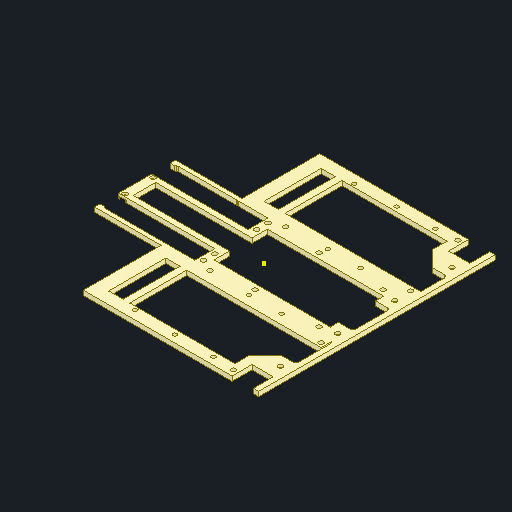
# Autodesk Inventor part: base
Saved by Autodesk Inventor 2023 (Build 270158000, 158)
## iProperties
Created: 2024-04-29
Part Number: base
Material: Nylon 6/6
Document SubType Name: Modeling
Designer: szymo
Density: 1.13 g/cm^3
Appearance: Nylon 6
Mass: 38.5341 g
Surface Area: 286.672 cm^2
Volume: 34.1009 cm^3
Author: szymo
Autodesk Inventor part; units mm, degrees
ref_plane "YZ Plane" through (0, 0, 0) normal (1, 0, 0) x (0, 1, 0)
ref_plane "XZ Plane" through (0, 0, 0) normal (0, 1, 0) x (-1, 0, 0)
ref_plane "XY Plane" through (0, 0, 0) normal (0, 0, 1) x (1, 0, 0)
sketch "Sketch1" plane through (0, 0, 0) normal (0, 1, 0) x (-1, 0, 0)
  line L0 (99, 89) -> (-99, 89)
  line L1 (-99, 89) -> (-99, -89)
  line L2 (-99, -89) -> (99, -89)
  line L3 (99, -89) -> (99, 89)
  line L4 (99, 89) -> (-99, -89) construction
  line L5 (-99, 89) -> (99, -89) construction
  line L6 (-99, 89) -> (-85, 89)
  line L7 (-85, 89) -> (-85, -89)
  line L8 (-85, -89) -> (-99, -89)
  line L9 (-99, -89) -> (-99, 89)
  line L10 (99, 89) -> (97, 89)
  line L11 (97, 89) -> (97, -89)
  line L12 (97, -89) -> (99, -89)
  line L13 (99, -89) -> (99, 89)
  line L14 (97, 33) -> (97, 35)
  line L15 (97, -33) -> (97, -35)
  line L16 (97, 32.8) -> (97, 35)
  line L17 (97, -32.8) -> (97, -35)
  line L18 (97, 89) -> (47, 89)
  line L19 (47, 89) -> (47, 30.5)
  line L20 (47, 30.5) -> (97, 30.5)
  line L21 (97, 30.5) -> (97, 89)
  line L22 (97, -89) -> (47, -89)
  line L23 (47, -89) -> (47, -30.5)
  line L24 (47, -30.5) -> (97, -30.5)
  line L25 (97, -30.5) -> (97, -89)
  line L26 (-81, 74) -> (-81, 89) projected
  line L27 (-81, 31) -> (-81, 55) projected
  line L28 (-81, -12) -> (-81, 12) projected
  line L29 (-81, -55) -> (-81, -31) projected
  line L30 (-81, -89) -> (-81, -74) projected
  arc A0 (-81, 74) -> (-79, 72) centre (-79, 74) ccw projected
  line L31 (-70, 72) -> (-79, 72) projected
  line L32 (-70, 57) -> (-70, 72) projected
  line L33 (-79, 57) -> (-70, 57) projected
  arc A1 (-79, 57) -> (-81, 55) centre (-79, 55) ccw projected
  arc A2 (-81, 31) -> (-79, 29) centre (-79, 31) ccw projected
  line L34 (-70, 29) -> (-79, 29) projected
  line L35 (-70, 14) -> (-70, 29) projected
  line L36 (-79, 14) -> (-70, 14) projected
  arc A3 (-79, 14) -> (-81, 12) centre (-79, 12) ccw projected
  arc A4 (-81, -12) -> (-79, -14) centre (-79, -12) ccw projected
  line L37 (-70, -14) -> (-79, -14) projected
  line L38 (-70, -29) -> (-70, -14) projected
  line L39 (-79, -29) -> (-70, -29) projected
  arc A5 (-79, -29) -> (-81, -31) centre (-79, -31) ccw projected
  arc A6 (-81, -55) -> (-79, -57) centre (-79, -55) ccw projected
  line L40 (-70, -57) -> (-79, -57) projected
  line L41 (-70, -72) -> (-70, -57) projected
  line L42 (-79, -72) -> (-70, -72) projected
  arc A7 (-79, -72) -> (-81, -74) centre (-79, -74) ccw projected
  circle A8 centre (-77, -64.5) radius 1.2295 projected
  circle A9 centre (-77, -21.5) radius 1.2295 projected
  circle A10 centre (-77, 21.5) radius 1.2295 projected
  circle A11 centre (-77, 64.5) radius 1.2295 projected
  line L43 (-65, 89) -> (-79, 89)
  line L44 (-79, 89) -> (-79, 75)
  line L45 (-79, 75) -> (-65, 75)
  line L46 (-65, 75) -> (-65, 89)
  line L47 (-65, 89) -> (-81, 89)
  line L48 (-81, 89) -> (-81, 74)
  line L49 (-81, 74) -> (-65, 74)
  line L50 (-65, 74) -> (-65, 89)
  line L51 (-99, 0) -> (97, 0)
  line L52 (0, 0) -> (-99, 0) construction
  line L53 (-65, -89) -> (-79, -89)
  line L54 (-79, -89) -> (-79, -75)
  line L55 (-79, -75) -> (-65, -75)
  line L56 (-65, -75) -> (-65, -89)
  line L57 (-65, -89) -> (-81, -89)
  line L58 (-81, -89) -> (-81, -74)
  line L59 (-81, -74) -> (-65, -74)
  line L60 (-65, -74) -> (-65, -89)
  line L61 (77.5, 29.5) -> (66.5, 29.5) projected
  line L62 (66.5, -29.5) -> (77.5, -29.5) projected
  point P0 (47, 89)
  point P1 (47, -89)
  point P2 (97, -30.5)
  point P3 (97, 30.5)
  point P4 (-81, -89)
  point P5 (-79, -74)
  dimension "d0" = 198
  dimension "d1" = 178
  dimension "d2" = 14
  dimension "d3" = 2
  dimension "d16" = 50
  dimension "d17" = 58.5
  dimension "d18" = 50
  dimension "d19" = 58.5
  dimension "d22" = 14
  dimension "d23" = 14
  dimension "d24" = 2
  dimension "d25" = 1
  dimension "d26" = 2
  dimension "d87" = 1
  dimension "d88" = 1
  constraints: 88 end point, 14 parallel, 10 symmetric about line, 8 perpendicular, 8 point on line, 7 horizontal, 4 midpoint, 2 collinear
  measures "d0" distance of L2.end L1.end
  measures "d1" distance of L1.end L0.end
  measures "d2" distance of L7.end L8.end
  measures "d3" distance of L12.end L11.end
  measures "d16" distance of L20.end L19.end
  measures "d17" distance of L19.end L18.end
  measures "d18" distance of L23.end L24.end
  measures "d19" distance of L22.end L23.end
  measures "d22" distance of L45.end L44.end
  measures "d23" distance of L44.end L43.end
  measures "d24" distance between parallel lines of L26 L44
  measures "d25" distance between parallel lines of L45 L49
  measures "d26" distance between parallel lines of L31 L49
  measures "d87" distance between parallel lines of L20 L61
  measures "d88" distance between parallel lines of L24 L62
extrude "Extrusion1" add sketch "Sketch1" along normal blind 3.5 contours L19 L20 L11 L51 L28 A3 L36 L35 L34 A2 L27 A1 L33 L32 L31 A0 L49 L50 L46 L0 | L2 L56 L60 L59 A7 L42 L41 L40 A6 L29 A5 L39 L38 L37 A4 L28 L51 L11 L24 L23 | L26 A0 L31 L32 L33 A1 L27 A2 L34 L35 L36 A3 L28 L51 L7 L0 | L28 A4 L37 L38 L39 A5 L29 A6 L40 L41 L42 A7 L30 L2 L7 L51 | A8 | A9 | A10 | A11
sketch "Sketch9" plane through (0, 0, 0) normal (0, -1, 0) x (1, 0, 0)
  circle A0 centre (-94, -10.5) radius 1.4 projected
  circle A1 centre (-94, 10.5) radius 1.4 projected
  circle A2 centre (-21.25, -24.25) radius 1.8 projected
  circle A3 centre (-21.25, -15.75) radius 1.8 projected
  circle A4 centre (-21.25, 15.75) radius 1.8 projected
  circle A5 centre (-21.25, 24.25) radius 1.8 projected
  circle A6 centre (-12.1414, 28.5) radius 1.8 projected
  circle A7 centre (-12.1414, -28.5) radius 1.8 projected
  circle A8 centre (17.4, -24.1) radius 1.6 projected
  circle A9 centre (17.4, 24.1) radius 1.6 projected
  circle A10 centre (65.6, 24.1) radius 1.6 projected
  circle A11 centre (65.6, -24.1) radius 1.6 projected
  circle A12 centre (76.75, -33.75) radius 1.8 projected
  circle A13 centre (76.75, 33.75) radius 1.8 projected
  circle A14 centre (61.5, 84.5) radius 1.8 projected
  circle A15 centre (61.5, -84.5) radius 1.8 projected
  point P0 (0, 0)
  constraints: 16 coincident
hole "m3" at (-94, 0, -10.5) at (-94, 0, 10.5) at (61.5, 0, -84.5) at (61.5, 0, 84.5) at (76.75, 0, 33.75) at (65.6, 0, 24.1) at (65.6, 0, -24.1) at (76.75, 0, -33.75) at (17.4, 0, 24.1) at (17.4, 0, -24.1) at (-12.1414, 0, -28.5) at (-21.25, 0, -24.25) at (-21.25, 0, -15.75) at (-21.25, 0, 15.75) at (-21.25, 0, 24.25) at (-12.1414, 0, 28.5) direction (0, 1, 0) diameter 3.6 end through all counterbore diameter 11 counterbore depth 0 clearance for "Hex Head Cap Screw ISO 24014 (Spotface)" size "M3" standard "ISO"
sketch "Sketch10" plane through (0, 0, 0) normal (0, -1, 0) x (1, 0, 0)
  circle A0 centre (61.5, -84.5) radius 1.8 projected
  circle A1 centre (76.75, -33.75) radius 1.8 projected
  circle A2 centre (65.6, -24.1) radius 1.8 projected
  circle A3 centre (65.6, 24.1) radius 1.8 projected
  circle A4 centre (76.75, 33.75) radius 1.8 projected
  circle A5 centre (61.5, 84.5) radius 1.8 projected
  circle A6 centre (17.4, 24.1) radius 1.8 projected
  circle A7 centre (17.4, -24.1) radius 1.8 projected
  circle A8 centre (-12.1414, -28.5) radius 1.8 projected
  circle A9 centre (-21.25, -24.25) radius 1.8 projected
  circle A10 centre (-21.25, -15.75) radius 1.8 projected
  circle A11 centre (-21.25, 15.75) radius 1.8 projected
  circle A12 centre (-21.25, 24.25) radius 1.8 projected
  circle A13 centre (-12.1414, 28.5) radius 1.8 projected
  circle A14 centre (-94, 10.5) radius 1.8 projected
  circle A15 centre (-94, -10.5) radius 1.8 projected
  line L0 (-94, -7.2668) -> (-91.2, -8.8834)
  line L1 (-91.2, -8.8834) -> (-91.2, -12.1166)
  line L2 (-91.2, -12.1166) -> (-94, -13.7332)
  line L3 (-94, -13.7332) -> (-96.8, -12.1166)
  line L4 (-96.8, -12.1166) -> (-96.8, -8.8834)
  line L5 (-96.8, -8.8834) -> (-94, -7.2668)
  line L6 (-94, 13.7332) -> (-91.2, 12.1166)
  line L7 (-91.2, 12.1166) -> (-91.2, 8.8834)
  line L8 (-91.2, 8.8834) -> (-94, 7.2668)
  line L9 (-94, 7.2668) -> (-96.8, 8.8834)
  line L10 (-96.8, 8.8834) -> (-96.8, 12.1166)
  line L11 (-96.8, 12.1166) -> (-94, 13.7332)
  point P0 (0, 0)
  dimension "d96" = 5.6
  dimension "d98" = 5.6
  constraints: 24 end point, 2 coincident, 26 other
  measures "d96" distance between parallel lines of L4 L1
  measures "d98" distance between parallel lines of L7 L10
extrude "m3_nut" cut sketch "Sketch10" against normal blind 1.6 contours L0 L1 L2 L3 L4 L5 | L6 L7 L8 L9 L10 L11
sketch "Sketch11" plane through (0, 0, 0) normal (0, -1, 0) x (1, 0, 0)
  circle A0 centre (-14.5, -82.4087) radius 1.15 projected
  circle A1 centre (16.5, -83.5) radius 1.15 projected
  circle A2 centre (45.4385, -83.5) radius 1.15 projected
  circle A3 centre (45.4385, 83.5) radius 1.15 projected
  circle A4 centre (16.5, 83.5) radius 1.15 projected
  circle A5 centre (-14.5, 82.4087) radius 1.15 projected
  circle A6 centre (18.4119, 29.75) radius 1.55 projected
  circle A7 centre (43.009, 29.75) radius 1.55 projected
  circle A8 centre (43.009, -29.75) radius 1.55 projected
  circle A9 centre (18.4119, -29.75) radius 1.55 projected
  point P0 (0, 0)
  constraints: 10 coincident
hole "m2.5" at (-14.5, 0, -82.4087) at (-14.5, 0, 82.4087) at (16.5, 0, 83.5) at (45.4385, 0, 83.5) at (43.009, 0, 29.75) at (18.4119, 0, 29.75) at (18.4119, 0, -29.75) at (43.009, 0, -29.75) at (45.4385, 0, -83.5) at (16.5, 0, -83.5) direction (0, 1, 0) diameter 3.1 end through all clearance for "Countersunk Flat Head Screw ISO 2009/7046" size "M2.5" standard "ISO"
sketch "m2.5_nut" plane through (0, 0, 0) normal (0, -1, 0) x (1, 0, 0)
  circle A0 centre (-14.5, -82.4087) radius 1.55 projected
  circle A1 centre (16.5, -83.5) radius 1.55 projected
  circle A2 centre (45.4385, -83.5) radius 1.55 projected
  circle A3 centre (45.4385, 83.5) radius 1.55 projected
  circle A4 centre (16.5, 83.5) radius 1.55 projected
  circle A5 centre (-14.5, 82.4087) radius 1.55 projected
  circle A6 centre (18.4119, -29.75) radius 1.55 projected
  circle A7 centre (43.009, -29.75) radius 1.55 projected
  circle A8 centre (43.009, 29.75) radius 1.55 projected
  circle A9 centre (18.4119, 29.75) radius 1.55 projected
  point P0 (0, 0)
sketch "Sketch13" plane through (0, 0, 0) normal (0, -1, 0) x (1, 0, 0)
  circle A0 centre (77, 21.5) radius 1.2295 projected
  circle A1 centre (77, -64.5) radius 1.2295 projected
  circle A2 centre (77, -21.5) radius 1.2295 projected
  circle A3 centre (77, 64.5) radius 1.2295 projected
  line L0 (79, -72) -> (70, -72) projected
  line L1 (70, -72) -> (70, -57) projected
  line L2 (70, -57) -> (79, -57) projected
  arc A4 (79, -57) -> (81, -55) centre (79, -55) ccw projected
  line L3 (81, -55) -> (81, -31) projected
  arc A5 (81, -31) -> (79, -29) centre (79, -31) ccw projected
  line L4 (79, -29) -> (70, -29) projected
  line L5 (70, -29) -> (70, -14) projected
  line L6 (70, -14) -> (79, -14) projected
  arc A6 (79, -14) -> (81, -12) centre (79, -12) ccw projected
  line L7 (81, -12) -> (81, 12) projected
  arc A7 (81, 12) -> (79, 14) centre (79, 12) ccw projected
  line L8 (79, 14) -> (70, 14) projected
  line L9 (70, 14) -> (70, 29) projected
  line L10 (70, 29) -> (79, 29) projected
  arc A8 (79, 29) -> (81, 31) centre (79, 31) ccw projected
  line L11 (81, 31) -> (81, 55) projected
  arc A9 (81, 55) -> (79, 57) centre (79, 55) ccw projected
  line L12 (79, 57) -> (70, 57) projected
  line L13 (70, 57) -> (70, 72) projected
  line L14 (70, 72) -> (79, 72) projected
  arc A10 (79, 72) -> (81, 74) centre (79, 74) ccw projected
  line L15 (81, 74) -> (81, 89) projected
  line L16 (85, 89) -> (81, 89) projected
  line L17 (85, -89) -> (85, 89) projected
  line L18 (85, -89) -> (81, -89) projected
  line L19 (81, -89) -> (81, -74) projected
  arc A11 (81, -74) -> (79, -72) centre (79, -74) ccw projected
  point P0 (0, 0)
  constraints: 4 coincident
hole "Hole6" at (77, 0, -64.5) at (77, 0, -21.5) at (77, 0, 21.5) at (77, 0, 64.5) direction (0, 1, 0) diameter 3.6 end through all countersink diameter 7 countersink angle 90
sketch "Sketch14" plane through (0, 3.5, 0) normal (0, -1, 0) x (1, 0, 0)
  circle A0 centre (70, -83) radius 1.75
  line L0 (14.0482, -86) -> (-12.0482, -86)
  arc A1 (-12.0482, -86) -> (-12, -85.6932) centre (-13, -85.6932) ccw
  line L1 (-12, -85.6932) -> (-12, -80.9087)
  arc A2 (-12, -80.9087) -> (-13, -79.9087) centre (-13, -80.9087) ccw
  line L2 (-13, -79.9087) -> (-16, -79.9087)
  arc A3 (-16, -79.9087) -> (-17, -80.9087) centre (-16, -80.9087) ccw
  line L3 (-17, -80.9087) -> (-17, -86)
  line L4 (-17, -86) -> (-21.8397, -86)
  arc A4 (-22.8397, -85) -> (-21.8397, -86) centre (-21.8397, -85) ccw
  line L5 (-22.8397, -85) -> (-22.8397, -81.6)
  line L6 (-22.8397, -81.6) -> (-31.5, -81.6)
  line L7 (-31.5, -81.6) -> (-40.1603, -81.6)
  line L8 (-40.1603, -85) -> (-40.1603, -81.6)
  arc A5 (-41.1603, -86) -> (-40.1603, -85) centre (-41.1603, -85) ccw
  line L9 (-41.1603, -86) -> (-47, -86)
  line L10 (-47, -89) -> (-47, -86)
  line L11 (-47, -89) -> (80, -89)
  line L12 (80, -89) -> (80, -88)
  line L13 (80, -88) -> (78.75, -88)
  arc A6 (74.5, -83.75) -> (78.75, -88) centre (78.75, -83.75) ccw
  line L14 (74.5, -83.75) -> (74.5, -80.25)
  arc A7 (74.5, -80.25) -> (70.25, -76) centre (70.25, -80.25) ccw
  line L15 (70.25, -76) -> (68.2269, -76)
  line L16 (68.2269, -76) -> (68.2269, -75.875)
  arc A8 (65, -71.75) -> (68.2269, -75.875) centre (69.25, -71.75) ccw
  line L17 (65, -71.75) -> (65, -69)
  line L18 (65, -69) -> (58, -69)
  line L19 (58, -69) -> (58, -74)
  line L20 (58, -74) -> (58, -86)
  line L21 (58, -86) -> (47.8903, -86)
  arc A9 (47.8903, -86) -> (47.9385, -85.6932) centre (46.9385, -85.6932) ccw
  line L22 (47.9385, -85.6932) -> (47.9385, -82)
  arc A10 (47.9385, -82) -> (46.9385, -81) centre (46.9385, -82) ccw
  line L23 (46.9385, -81) -> (43.9385, -81)
  arc A11 (43.9385, -81) -> (42.9385, -82) centre (43.9385, -82) ccw
  line L24 (42.9385, -82) -> (42.9385, -85.6932)
  arc A12 (42.9385, -85.6932) -> (42.9867, -86) centre (43.9385, -85.6932) ccw
  line L25 (42.9867, -86) -> (18.9518, -86)
  arc A13 (18.9518, -86) -> (19, -85.6932) centre (18, -85.6932) ccw
  line L26 (19, -85.6932) -> (19, -82)
  arc A14 (19, -82) -> (18, -81) centre (18, -82) ccw
  line L27 (18, -81) -> (15, -81)
  arc A15 (15, -81) -> (14, -82) centre (15, -82) ccw
  line L28 (14, -82) -> (14, -85.6932)
  arc A16 (14, -85.6932) -> (14.0482, -86) centre (15, -85.6932) ccw
  circle A17 centre (16.5, -83.5) radius 1.15
  circle A18 centre (-14.5, -82.4087) radius 1.15
  circle A19 centre (45.4385, -83.5) radius 1.15
  circle A20 centre (61.5, -84.5) radius 1.8
  circle A21 centre (18.4119, -29.75) radius 1.55
  circle A22 centre (43.009, -29.75) radius 1.55
  circle A23 centre (17.4, -24.1) radius 1.6
  circle A24 centre (65.6, -24.1) radius 1.6
  circle A25 centre (-12.1414, -28.5) radius 1.8
  circle A26 centre (76.75, -33.75) radius 1.8
  arc A27 (69.6, -27.9275) -> (73.5136, -30.785) centre (72.6, -27.9275) ccw
  line L29 (69.6, -27.9275) -> (69.6, -20.1)
  line L30 (69.6, -20.1) -> (61.6, -20.1)
  line L31 (61.6, -20.1) -> (61.6, -27)
  arc A28 (56.6, -32) -> (61.6, -27) centre (56.6, -27) ccw
  line L32 (56.6, -32) -> (53.1217, -32)
  arc A29 (47.3676, -27.7) -> (53.1217, -32) centre (53.1217, -26) ccw
  line L33 (47.3676, -27.7) -> (38.6504, -27.7)
  arc A30 (32.8963, -32) -> (38.6504, -27.7) centre (32.8963, -26) ccw
  line L34 (32.8963, -32) -> (28.5247, -32)
  arc A31 (22.7705, -27.7) -> (28.5247, -32) centre (28.5247, -26) ccw
  line L35 (22.7705, -27.7) -> (22.7705, -20.1)
  line L36 (22.7705, -20.1) -> (14.0533, -20.1)
  line L37 (14.0533, -20.1) -> (14.0533, -27.7)
  arc A32 (8.2992, -32) -> (14.0533, -27.7) centre (8.2992, -26) ccw
  line L38 (8.2992, -32) -> (-0.7828, -32)
  arc A33 (-7.7828, -25) -> (-0.7828, -32) centre (-0.7828, -25) ccw
  line L39 (-7.7828, -25) -> (-16.5, -25)
  line L40 (-16.5, -28) -> (-16.5, -25)
  arc A34 (-20.5, -32) -> (-16.5, -28) centre (-20.5, -28) ccw
  line L41 (-20.5, -32) -> (-47, -32)
  line L42 (-47, -37) -> (-47, -32)
  line L43 (-47, -37) -> (52.4519, -37)
  line L44 (52.4519, -36) -> (52.4519, -37)
  line L45 (52.4519, -37) -> (80, -37)
  line L46 (80, -37) -> (80, -30.5)
  line L47 (80, -30.5) -> (75.3408, -30.5)
  arc A35 (75.3408, -30.5) -> (73.5136, -30.785) centre (75.3408, -36.5) ccw
  circle A36 centre (18.4119, 29.75) radius 1.55
  circle A37 centre (43.009, 29.75) radius 1.55
  circle A38 centre (17.4, 24.1) radius 1.6
  circle A39 centre (65.6, 24.1) radius 1.6
  circle A40 centre (-12.1414, 28.5) radius 1.8
  circle A41 centre (76.75, 33.75) radius 1.8
  arc A42 (73.5136, 30.785) -> (69.6, 27.9275) centre (72.6, 27.9275) ccw
  arc A43 (73.5136, 30.785) -> (75.3408, 30.5) centre (75.3408, 36.5) ccw
  line L48 (80, 30.5) -> (75.3408, 30.5)
  line L49 (80, 37) -> (80, 30.5)
  line L50 (52.4519, 37) -> (80, 37)
  line L51 (52.4519, 36) -> (52.4519, 37)
  line L52 (-47, 37) -> (52.4519, 37)
  line L53 (-47, 37) -> (-47, 32)
  line L54 (-20.5, 32) -> (-47, 32)
  arc A44 (-16.5, 28) -> (-20.5, 32) centre (-20.5, 28) ccw
  line L55 (-16.5, 28) -> (-16.5, 25)
  line L56 (-7.7828, 25) -> (-16.5, 25)
  arc A45 (-0.7828, 32) -> (-7.7828, 25) centre (-0.7828, 25) ccw
  line L57 (8.2992, 32) -> (-0.7828, 32)
  arc A46 (14.0533, 27.7) -> (8.2992, 32) centre (8.2992, 26) ccw
  line L58 (14.0533, 20.1) -> (14.0533, 27.7)
  line L59 (22.7705, 20.1) -> (14.0533, 20.1)
  line L60 (22.7705, 27.7) -> (22.7705, 20.1)
  arc A47 (28.5247, 32) -> (22.7705, 27.7) centre (28.5247, 26) ccw
  line L61 (32.8963, 32) -> (28.5247, 32)
  arc A48 (38.6504, 27.7) -> (32.8963, 32) centre (32.8963, 26) ccw
  line L62 (47.3676, 27.7) -> (38.6504, 27.7)
  arc A49 (53.1217, 32) -> (47.3676, 27.7) centre (53.1217, 26) ccw
  line L63 (56.6, 32) -> (53.1217, 32)
  arc A50 (61.6, 27) -> (56.6, 32) centre (56.6, 27) ccw
  line L64 (61.6, 20.1) -> (61.6, 27)
  line L65 (69.6, 20.1) -> (61.6, 20.1)
  line L66 (69.6, 27.9275) -> (69.6, 20.1)
  line L67 (14.0482, 86) -> (-12.0482, 86)
  arc A51 (14.0482, 86) -> (14, 85.6932) centre (15, 85.6932) ccw
  line L68 (14, 82) -> (14, 85.6932)
  arc A52 (14, 82) -> (15, 81) centre (15, 82) ccw
  line L69 (18, 81) -> (15, 81)
  arc A53 (18, 81) -> (19, 82) centre (18, 82) ccw
  line L70 (19, 85.6932) -> (19, 82)
  arc A54 (19, 85.6932) -> (18.9518, 86) centre (18, 85.6932) ccw
  line L71 (42.9867, 86) -> (18.9518, 86)
  arc A55 (42.9867, 86) -> (42.9385, 85.6932) centre (43.9385, 85.6932) ccw
  line L72 (42.9385, 82) -> (42.9385, 85.6932)
  arc A56 (42.9385, 82) -> (43.9385, 81) centre (43.9385, 82) ccw
  line L73 (46.9385, 81) -> (43.9385, 81)
  arc A57 (46.9385, 81) -> (47.9385, 82) centre (46.9385, 82) ccw
  line L74 (47.9385, 85.6932) -> (47.9385, 82)
  arc A58 (47.9385, 85.6932) -> (47.8903, 86) centre (46.9385, 85.6932) ccw
  line L75 (58, 86) -> (47.8903, 86)
  line L76 (58, 74) -> (58, 86)
  line L77 (58, 69) -> (58, 74)
  line L78 (65, 69) -> (58, 69)
  line L79 (65, 71.75) -> (65, 69)
  arc A59 (68.2269, 75.875) -> (65, 71.75) centre (69.25, 71.75) ccw
  line L80 (68.2269, 76) -> (68.2269, 75.875)
  line L81 (70.25, 76) -> (68.2269, 76)
  arc A60 (70.25, 76) -> (74.5, 80.25) centre (70.25, 80.25) ccw
  line L82 (74.5, 83.75) -> (74.5, 80.25)
  arc A61 (78.75, 88) -> (74.5, 83.75) centre (78.75, 83.75) ccw
  line L83 (80, 88) -> (78.75, 88)
  line L84 (80, 89) -> (80, 88)
  line L85 (-47, 89) -> (80, 89)
  line L86 (-47, 89) -> (-47, 86)
  line L87 (-41.1603, 86) -> (-47, 86)
  arc A62 (-40.1603, 85) -> (-41.1603, 86) centre (-41.1603, 85) ccw
  line L88 (-40.1603, 85) -> (-40.1603, 81.6)
  line L89 (-31.5, 81.6) -> (-40.1603, 81.6)
  line L90 (-22.8397, 81.6) -> (-31.5, 81.6)
  line L91 (-22.8397, 85) -> (-22.8397, 81.6)
  arc A63 (-21.8397, 86) -> (-22.8397, 85) centre (-21.8397, 85) ccw
  line L92 (-17, 86) -> (-21.8397, 86)
  line L93 (-17, 80.9087) -> (-17, 86)
  arc A64 (-17, 80.9087) -> (-16, 79.9087) centre (-16, 80.9087) ccw
  line L94 (-13, 79.9087) -> (-16, 79.9087)
  arc A65 (-13, 79.9087) -> (-12, 80.9087) centre (-13, 80.9087) ccw
  line L95 (-12, 85.6932) -> (-12, 80.9087)
  arc A66 (-12, 85.6932) -> (-12.0482, 86) centre (-13, 85.6932) ccw
  circle A67 centre (16.5, 83.5) radius 1.15
  circle A68 centre (-14.5, 82.4087) radius 1.15
  circle A69 centre (45.4385, 83.5) radius 1.15
  circle A70 centre (70, 80) radius 1.75
  circle A71 centre (61.5, 84.5) radius 1.8
  line L96 (-24.5, 21) -> (-24.5, 27.5)
  line L97 (-18, 21) -> (-24.5, 21)
  line L98 (-18, 30.5) -> (-18, 21)
  line L99 (-97, 30.5) -> (-18, 30.5)
  line L100 (-97, 30.5) -> (-97, 26.5)
  line L101 (-93.7321, 26.5) -> (-97, 26.5)
  arc A72 (-93.7321, 26.5) -> (-92.866, 27) centre (-93.7321, 27.5) ccw
  arc A73 (-92, 27.5) -> (-92.866, 27) centre (-92, 26.5) ccw
  line L102 (-78.8409, 27.5) -> (-92, 27.5)
  spline S0 degree 3 poles (-75.7417, 26) (-75.7753, 26.0631) (-75.8128, 26.1246) (-76.0566, 26.4695) (-76.3938, 26.7337) (-77.0078, 27.0936) (-77.4015, 27.2556) (-78.0794, 27.4407) (-78.4928, 27.5) (-78.8409, 27.5) knots 0 0 0 0 0.058061 0.058061 0.375369 0.375369 0.690666 0.690666 1 1 1 1
  line L103 (-68.2583, 26) -> (-75.7417, 26)
  spline S1 degree 3 poles (-68.2583, 26) (-68.2382, 26.0379) (-68.2174, 26.0746) (-68.0344, 26.3642) (-67.7636, 26.6069) (-67.1915, 26.9981) (-66.7665, 27.1943) (-66.018, 27.4248) (-65.5523, 27.5) (-65.1591, 27.5) knots 0 0 0 0 0.035027 0.035027 0.30423 0.30423 0.650773 0.650773 1 1 1 1
  line L104 (-47.8217, 27.5) -> (-65.1591, 27.5)
  spline S2 degree 3 poles (-45.6477, 26) (-45.6733, 26.0786) (-45.7018, 26.1547) (-45.8425, 26.4593) (-46.0302, 26.7067) (-46.4247, 27.0666) (-46.7063, 27.2391) (-47.2204, 27.4381) (-47.5457, 27.5) (-47.8217, 27.5) knots 0 0 0 0 0.086487 0.086487 0.378353 0.378353 0.688736 0.688736 1 1 1 1
  line L105 (-38.9709, 26) -> (-45.6477, 26)
  spline S3 degree 3 poles (-38.9709, 26) (-38.9452, 26.0786) (-38.9168, 26.1547) (-38.7761, 26.4593) (-38.5883, 26.7067) (-38.1939, 27.0666) (-37.9122, 27.2391) (-37.3982, 27.4381) (-37.0728, 27.5) (-36.7968, 27.5) knots 0 0 0 0 0.086487 0.086487 0.378353 0.378353 0.688736 0.688736 1 1 1 1
  line L106 (-24.5, 27.5) -> (-36.7968, 27.5)
  circle A74 centre (-21.25, 24.25) radius 1.8
  circle A75 centre (-94, 10.5) radius 1.4
  circle A76 centre (-21.25, 15.75) radius 1.8
  line L107 (-37.4639, 12.5) -> (-24, 12.5)
  spline S4 degree 3 poles (-38.9709, 13) (-38.7801, 12.8633) (-38.5578, 12.7418) (-38.085, 12.5634) (-37.7489, 12.5) (-37.4639, 12.5) knots 0 0 0 0 0.435873 0.435873 1 1 1 1
  line L108 (-38.9709, 13) -> (-41.358, 13)
  spline S5 degree 3 poles (-43.2606, 13) (-43.1675, 13) (-43.0559, 12.9938) (-42.7588, 12.9716) (-42.5141, 12.9484) (-42.1044, 12.9484) (-41.8597, 12.9716) (-41.5626, 12.9938) (-41.4511, 13) (-41.358, 13) knots 0 0 0 0 0.156235 0.156235 0.5 0.5 0.843765 0.843765 1 1 1 1
  line L109 (-43.2606, 13) -> (-45.6477, 13)
  spline S6 degree 3 poles (-45.6477, 13) (-45.8385, 12.8633) (-46.0608, 12.7418) (-46.5335, 12.5634) (-46.8696, 12.5) (-47.1547, 12.5) knots 0 0 0 0 0.435873 0.435873 1 1 1 1
  line L110 (-67.6471, 12.5) -> (-47.1547, 12.5)
  line L111 (-70.9629, 12.5) -> (-67.6471, 12.5)
  line L112 (-72, 12.5) -> (-70.9629, 12.5)
  line L113 (-73.0371, 12.5) -> (-72, 12.5)
  line L114 (-76.3529, 12.5) -> (-73.0371, 12.5)
  line L115 (-97, 12.5) -> (-76.3529, 12.5)
  line L116 (-97, 8.5) -> (-97, 12.5)
  line L117 (-97, 8.5) -> (-17.5, 8.5)
  line L118 (-17.5, 8.5) -> (-17.5, 19)
  line L119 (-24, 19) -> (-17.5, 19)
  line L120 (-24, 12.5) -> (-24, 19)
  circle A77 centre (-94, -10.5) radius 1.4
  circle A78 centre (-21.25, -15.75) radius 1.8
  line L121 (-37.4639, -12.5) -> (-24, -12.5)
  line L122 (-24, -12.5) -> (-24, -19)
  line L123 (-24, -19) -> (-17.5, -19)
  line L124 (-17.5, -8.5) -> (-17.5, -19)
  line L125 (-97, -8.5) -> (-17.5, -8.5)
  line L126 (-97, -8.5) -> (-97, -12.5)
  line L127 (-97, -12.5) -> (-76.3529, -12.5)
  line L128 (-76.3529, -12.5) -> (-73.0371, -12.5)
  line L129 (-73.0371, -12.5) -> (-72, -12.5)
  line L130 (-72, -12.5) -> (-70.9629, -12.5)
  line L131 (-70.9629, -12.5) -> (-67.6471, -12.5)
  line L132 (-67.6471, -12.5) -> (-47.1547, -12.5)
  spline S7 degree 3 poles (-45.6477, -13) (-45.8385, -12.8633) (-46.0608, -12.7418) (-46.5335, -12.5634) (-46.8696, -12.5) (-47.1547, -12.5) knots 0 0 0 0 0.435873 0.435873 1 1 1 1
  line L133 (-43.2606, -13) -> (-45.6477, -13)
  spline S8 degree 3 poles (-43.2606, -13) (-43.1675, -13) (-43.0559, -12.9938) (-42.7588, -12.9716) (-42.5141, -12.9484) (-42.1044, -12.9484) (-41.8597, -12.9716) (-41.5626, -12.9938) (-41.4511, -13) (-41.358, -13) knots 0 0 0 0 0.156235 0.156235 0.5 0.5 0.843765 0.843765 1 1 1 1
  line L134 (-38.9709, -13) -> (-41.358, -13)
  spline S9 degree 3 poles (-38.9709, -13) (-38.7801, -12.8633) (-38.5578, -12.7418) (-38.085, -12.5634) (-37.7489, -12.5) (-37.4639, -12.5) knots 0 0 0 0 0.435873 0.435873 1 1 1 1
  line L135 (-24.5, -21) -> (-24.5, -27.5)
  line L136 (-24.5, -27.5) -> (-36.7968, -27.5)
  spline S10 degree 3 poles (-38.9709, -26) (-38.9452, -26.0786) (-38.9168, -26.1547) (-38.7761, -26.4593) (-38.5883, -26.7067) (-38.1939, -27.0666) (-37.9122, -27.2391) (-37.3982, -27.4381) (-37.0728, -27.5) (-36.7968, -27.5) knots 0 0 0 0 0.086487 0.086487 0.378353 0.378353 0.688736 0.688736 1 1 1 1
  line L137 (-38.9709, -26) -> (-45.6477, -26)
  spline S11 degree 3 poles (-45.6477, -26) (-45.6733, -26.0786) (-45.7018, -26.1547) (-45.8425, -26.4593) (-46.0302, -26.7067) (-46.4247, -27.0666) (-46.7063, -27.2391) (-47.2204, -27.4381) (-47.5457, -27.5) (-47.8217, -27.5) knots 0 0 0 0 0.086487 0.086487 0.378353 0.378353 0.688736 0.688736 1 1 1 1
  line L138 (-47.8217, -27.5) -> (-65.1591, -27.5)
  spline S12 degree 3 poles (-68.2583, -26) (-68.2382, -26.0379) (-68.2174, -26.0746) (-68.0344, -26.3642) (-67.7636, -26.6069) (-67.1915, -26.9981) (-66.7665, -27.1943) (-66.018, -27.4248) (-65.5523, -27.5) (-65.1591, -27.5) knots 0 0 0 0 0.035027 0.035027 0.30423 0.30423 0.650773 0.650773 1 1 1 1
  line L139 (-68.2583, -26) -> (-75.7417, -26)
  spline S13 degree 3 poles (-75.7417, -26) (-75.7753, -26.0631) (-75.8128, -26.1246) (-76.0566, -26.4695) (-76.3938, -26.7337) (-77.0078, -27.0936) (-77.4015, -27.2556) (-78.0794, -27.4407) (-78.4928, -27.5) (-78.8409, -27.5) knots 0 0 0 0 0.058061 0.058061 0.375369 0.375369 0.690666 0.690666 1 1 1 1
  line L140 (-78.8409, -27.5) -> (-92, -27.5)
  arc A79 (-92.866, -27) -> (-92, -27.5) centre (-92, -26.5) ccw
  arc A80 (-92.866, -27) -> (-93.7321, -26.5) centre (-93.7321, -27.5) ccw
  line L141 (-93.7321, -26.5) -> (-97, -26.5)
  line L142 (-97, -30.5) -> (-97, -26.5)
  line L143 (-97, -30.5) -> (-18, -30.5)
  line L144 (-18, -30.5) -> (-18, -21)
  line L145 (-18, -21) -> (-24.5, -21)
  circle A81 centre (-21.25, -24.25) radius 1.8
  line L146 (-22, -8.5) -> (-22, 8.5)
  line L147 (-22, 8.5) -> (-90, 8.5)
  line L148 (-90, 8.5) -> (-90, -8.5)
  line L149 (-90, -8.5) -> (-22, -8.5)
  line L150 (-15.5, -70.1149) -> (50.5, -70.1149)
  line L151 (50.5, -70.1149) -> (50.5, -40.1149)
  line L152 (-15.5, -40.1149) -> (50.5, -40.1149)
  line L153 (-15.5, -70.1149) -> (-15.5, -40.1149)
  line L154 (50.5, 71.1831) -> (-15.5, 71.1831)
  line L155 (-15.5, 71.1831) -> (-15.5, 41.1831)
  line L156 (50.5, 41.1831) -> (-15.5, 41.1831)
  line L157 (50.5, 71.1831) -> (50.5, 41.1831)
  line L158 (-36.8852, -42) -> (-31.5, -42)
  line L159 (-31.5, -42) -> (-26.1148, -42)
  line L160 (-26.1148, -42) -> (-26.1148, -69.7)
  line L161 (-26.1148, -69.7) -> (-36.8852, -69.7)
  line L162 (-36.8852, -69.7) -> (-36.8852, -42)
  line L163 (-26.1148, 42) -> (-31.5, 42)
  line L164 (-31.5, 42) -> (-36.8852, 42)
  line L165 (-36.8852, 42) -> (-36.8852, 69.7)
  line L166 (-36.8852, 69.7) -> (-26.1148, 69.7)
  line L167 (-26.1148, 69.7) -> (-26.1148, 42)
  line L168 (85, -89) -> (99, -89)
  line L169 (99, -89) -> (99, 89)
  line L170 (85, 89) -> (99, 89)
  line L171 (85, -89) -> (85, 89)
  circle A82 centre (77, 21.5) radius 1.2295
  circle A83 centre (77, -64.5) radius 1.2295
  circle A84 centre (77, -21.5) radius 1.2295
  circle A85 centre (77, 64.5) radius 1.2295
  line L172 (70, -72) -> (79, -72)
  arc A86 (81, -74) -> (79, -72) centre (79, -74) ccw
  line L173 (81, -74) -> (81, -89)
  line L174 (81, -89) -> (85, -89)
  line L175 (85, -89) -> (85, 89)
  line L176 (81, 89) -> (85, 89)
  line L177 (81, 89) -> (81, 74)
  arc A87 (79, 72) -> (81, 74) centre (79, 74) ccw
  line L178 (79, 72) -> (70, 72)
  line L179 (70, 57) -> (70, 72)
  line L180 (70, 57) -> (79, 57)
  arc A88 (81, 55) -> (79, 57) centre (79, 55) ccw
  line L181 (81, 55) -> (81, 31)
  arc A89 (79, 29) -> (81, 31) centre (79, 31) ccw
  line L182 (79, 29) -> (70, 29)
  line L183 (70, 14) -> (70, 29)
  line L184 (70, 14) -> (79, 14)
  arc A90 (81, 12) -> (79, 14) centre (79, 12) ccw
  line L185 (81, 12) -> (81, -12)
  arc A91 (79, -14) -> (81, -12) centre (79, -12) ccw
  line L186 (79, -14) -> (70, -14)
  line L187 (70, -29) -> (70, -14)
  line L188 (70, -29) -> (79, -29)
  arc A92 (81, -31) -> (79, -29) centre (79, -31) ccw
  line L189 (81, -31) -> (81, -55)
  arc A93 (79, -57) -> (81, -55) centre (79, -55) ccw
  line L190 (79, -57) -> (70, -57)
  line L191 (70, -72) -> (70, -57)
  line L192 (81, -89) -> (81, -74)
  line L193 (81, -74) -> (65, -74)
  line L194 (65, -74) -> (65, -89)
  line L195 (65, 89) -> (65, 74)
  line L196 (65, 74) -> (81, 74)
  line L197 (81, 74) -> (81, 89)
  line L198 (70, -57) -> (58, -69)
  line L199 (70, 57) -> (58, 69)
  line L200 (58, 89) -> (-47, 89)
  line L201 (-47, 89) -> (-47, 79.9087)
  line L202 (-47, 79.9087) -> (58, 79.9087)
  line L203 (58, 79.9087) -> (58, 89)
  line L204 (58, -89) -> (-47, -89)
  line L205 (-47, -89) -> (-47, -79.9087)
  line L206 (-47, -79.9087) -> (58, -79.9087)
  line L207 (58, -79.9087) -> (58, -89)
  line L208 (81, -37) -> (-47, -37)
  line L209 (-47, -37) -> (-47, -20.1)
  line L210 (-47, -20.1) -> (81, -20.1)
  line L211 (81, -20.1) -> (81, -37)
  line L212 (80, 37) -> (-47, 37)
  line L213 (-47, 37) -> (-47, 20.1)
  line L214 (-47, 20.1) -> (80, 20.1)
  line L215 (80, 20.1) -> (80, 37)
  line L216 (-36.8852, -79.9087) -> (-41.8852, -79.9087)
  line L217 (-41.8852, -79.9087) -> (-41.8852, -36.5)
  line L218 (-41.8852, -36.5) -> (-36.8852, -36.5)
  line L219 (-36.8852, -36.5) -> (-36.8852, -79.9087)
  line L220 (-36.8852, 37) -> (-41.8852, 37)
  line L221 (-41.8852, 37) -> (-41.8852, 79.9087)
  line L222 (-41.8852, 79.9087) -> (-36.8852, 79.9087)
  line L223 (-36.8852, 79.9087) -> (-36.8852, 37)
  line L224 (-21.1148, -79.9087) -> (-26.1148, -79.9087)
  line L225 (-26.1148, -79.9087) -> (-26.1148, -37)
  line L226 (-26.1148, -37) -> (-21.1148, -37)
  line L227 (-21.1148, -37) -> (-21.1148, -79.9087)
  line L228 (-26.1148, 37) -> (-21.1148, 37)
  line L229 (-21.1148, 37) -> (-21.1148, 79.9087)
  line L230 (-21.1148, 79.9087) -> (-26.1148, 79.9087)
  line L231 (-26.1148, 79.9087) -> (-26.1148, 37)
  line L232 (-97, -30.5) -> (-17.5, -30.5)
  line L233 (-17.5, -30.5) -> (-17.5, -8.5)
  line L234 (-17.5, -8.5) -> (-97, -8.5)
  line L235 (-97, -8.5) -> (-97, -30.5)
  line L236 (-97, 30.5) -> (-17.5, 30.5)
  line L237 (-17.5, 30.5) -> (-17.5, 8.5)
  line L238 (-17.5, 8.5) -> (-97, 8.5)
  line L239 (-97, 8.5) -> (-97, 30.5)
  line L240 (-97, -30.5) -> (-47, -30.5)
  line L241 (-47, -30.5) -> (-47, -27.5)
  line L242 (-17.5, -27.5) -> (-97, -27.5)
  line L243 (-97, -27.5) -> (-97, -30.5)
  line L244 (-47, 30.5) -> (-97, 30.5)
  line L245 (-97, 30.5) -> (-97, 27.5)
  line L246 (-97, 27.5) -> (-17.5, 27.5)
  line L247 (-47, 27.5) -> (-47, 30.5)
  line L248 (-97, 8.5) -> (-24, 8.5)
  line L249 (-24, 8.5) -> (-24, 12.5)
  line L250 (-24, 12.5) -> (-97, 12.5)
  line L251 (-97, 12.5) -> (-97, 8.5)
  line L252 (-97, -8.5) -> (-24, -8.5)
  line L253 (-24, -8.5) -> (-24, -12.5)
  line L254 (-24, -12.5) -> (-97, -12.5)
  line L255 (-97, -12.5) -> (-97, -8.5)
  line L256 (-24.5, -27.5) -> (-24.5, -12.5)
  line L257 (-24.5, 27.5) -> (-24.5, 12.5)
  point P0 (0, 0)
  point P1 (-31.5, -37)
  point P2 (-31.5, 37)
  point P3 (-47, 27.5)
  point P4 (-47, 27.3523)
  point P5 (-47, -27.3523)
  point P6 (58, 79.9087)
  point P7 (80, 29.2679)
  point P8 (70, 20.1)
  point P9 (-17.5, 20.1)
  point P10 (-17.5, -20.1)
  point P11 (70, -20.1)
  point P12 (-26.1148, -37)
  point P13 (-36.8852, -37)
  dimension "d115" = 16.9
  dimension "d116" = 5
  dimension "d117" = 5
  dimension "d118" = 5
  dimension "d119" = 5
  constraints: 140 end point, 28 parallel, 25 point on line, 20 horizontal, 16 perpendicular, 15 collinear, 4 vertical, 12 other
  measures "d115" distance between parallel lines of L43 L210
  measures "d116" distance of L217.end L218.end
  measures "d117" distance of L221.end L222.end
  measures "d118" distance of L225.end L226.end
  measures "d119" distance of L230.end L229.end
extrude "Extrusion6" cut sketch "Sketch14" along normal blind 3.5 contours L2 L206 L227 L43 L45 L208 L189 A93 L190 L198 L19 L20 | L206 L219 L161 L225 | L161 L162 L158 L159 L160 | L225 L159 L158 L219 L43 | L210 L30 L36 L233 L124 L125 L146 L117 L118 L237 L214 L59 L65 L183 L184 A90 L185 A91 L186 L187 | L209 S11 L137 S10 L242 | L209 L210 L256 L135 L136 S10 L137 S11 | S11 L138 S12 L139 S13 L140 A79 A80 L141 L235 L127 L128 L129 L130 L131 L132 S7 L133 S8 L134 S9 L121 L256 L210 L209 | L242 S13 L139 S12 | L148 L117 L146 L125 | S9 L134 S8 L133 S7 L254 | L180 A88 L181 A89 L215 L49 L50 L52 L229 L202 L94 L76 L77 L199 | L239 L101 A72 A73 L102 S0 L103 S1 L104 S2 L213 L214 L257 L107 S4 L108 S5 L109 S6 L110 L111 L112 L113 L114 L115 | L250 S6 L109 S5 L108 S4 | L214 L213 S2 L105 S3 L106 L96 L257 | L202 L231 L166 L223 | L246 S1 L103 S0 | L213 L246 S3 L105 S2 | L166 L167 L163 L164 L165 | L223 L164 L163 L231 L52 | L153 L152 L151 L150 | L157 L156 L155 L154
body "Solid1"
